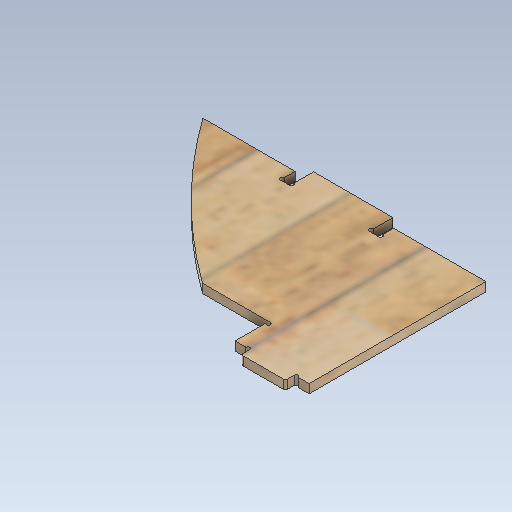
# Autodesk Inventor part: Support A1
Saved by Autodesk Inventor 2020 (Build 240168000, 168)
## iProperties
Created: 2020-03-07
Part Number: Support A1
Material: Wood (Maple)
Document SubType Name: Modeling
Designer: Daniel Wikman
Density: 0.67 g/cm^3
Appearance: Natural Maple - Glossy Dark Tint
Author: Daniel Wikman
Autodesk Inventor part; units mm, degrees
ref_plane "YZ Plane" through (0, 0, 0) normal (1, 0, 0) x (0, 1, 0)
ref_plane "XZ Plane" through (0, 0, 0) normal (0, 1, 0) x (-1, 0, 0)
ref_plane "XY Plane" through (0, 0, 0) normal (0, 0, 1) x (1, 0, 0)
sketch "Sketch1" plane through (0, 0, 0) normal (0, 1, 0) x (-1, 0, 0)
  arc A0 (-1.4864, -17.3614) -> (1.1787, -17.296) centre (-0.1546, -17.296) ccw
  arc A1 (31.1823, -17.2881) -> (33.847, -17.3614) centre (32.5157, -17.2881) ccw
  line L0 (33.847, -17.3614) -> (41.1803, -17.3614)
  line L1 (-1.4864, -17.3614) -> (-8.8197, -17.3614)
  line L2 (-8.8197, -17.3614) -> (-8.8197, -136.8614)
  line L3 (41.1803, -17.3614) -> (41.1803, -38.0281)
  arc A2 (41.1803, -38.0281) -> (40.0555, -40.0773) centre (40.0555, -38.7439) ccw
  line L4 (40.0555, -40.0773) -> (85.8888, -40.0773)
  line L5 (-8.8197, -136.8614) -> (53.5136, -136.8614)
  line L6 (53.5136, -136.8614) -> (53.5136, -129.5281)
  arc A3 (53.5136, -126.8614) -> (53.5136, -129.5281) centre (53.5136, -128.1947) ccw
  arc A4 (60.0136, -129.5281) -> (60.0136, -126.8614) centre (60.0136, -128.1947) ccw
  line L7 (60.0136, -129.5281) -> (60.0136, -142.8614)
  line L8 (60.0136, -126.8614) -> (53.5136, -126.8614)
  line L9 (120.137, -136.8614) -> (120.137, -129.5281)
  arc A5 (120.137, -129.5281) -> (120.137, -126.8614) centre (120.137, -128.1947) ccw
  arc A6 (113.637, -126.8614) -> (113.637, -129.5281) centre (113.637, -128.1947) ccw
  line L10 (113.637, -129.5281) -> (113.637, -142.8614)
  line L11 (113.637, -126.8614) -> (120.137, -126.8614)
  arc A7 (182.4703, -136.8614) -> (85.8888, -40.0773) centre (-162.7379, -384.7652) ccw
  line L12 (120.137, -136.8614) -> (182.4703, -136.8614)
  arc A8 (2.512, -11.3614) -> (1.1787, -12.6947) centre (2.512, -12.6947) ccw
  line L13 (1.1787, -12.6947) -> (1.1787, -17.296)
  arc A9 (31.1823, -12.6947) -> (29.849, -11.3614) centre (29.849, -12.6947) ccw
  line L14 (2.512, -11.3614) -> (29.849, -11.3614)
  line L15 (31.1823, -17.2881) -> (31.1823, -12.6947)
  line L16 (60.0136, -142.8614) -> (113.637, -142.8614)
  point P0 (0, 0)
  point P1 (28.8512, 3.0303)
  point P2 (-1.1488, 3.0309)
  dimension "d1" = 2.6667
  dimension "d2" = 30
  dimension "d4" = 2.6667
  dimension "d6" = 7.3333
  dimension "d7" = 7.3333
  dimension "d8" = 20.6667
  dimension "d9" = 2.6667
  dimension "d10" = 45.8333
  dimension "d11" = 119.5
  dimension "d12" = 62.3333
  dimension "d19" = 7.3333
  dimension "d53" = 2.6667
  dimension "d56" = 2.6667
  dimension "d58" = 6.5
  dimension "d59" = 13.3333
  dimension "d61" = 425
  dimension "d64" = 13.3333
  dimension "d67" = 7.3333
  dimension "d73" = 50
  dimension "d74" = 2.6667
  dimension "d75" = 6
  dimension "d76" = 191.29
  dimension "d77" = 6.5
  dimension "d78" = 6.5
  dimension "d79" = 6.5
  dimension "d80" = 1.3333
  dimension "d81" = 1.3333
  dimension "d82" = 90
  dimension "d83" = 2.6667
  dimension "d84" = 2.6667
  dimension "d85" = 2.6667
  dimension "d86" = 2.6667
  dimension "d87" = 53.6233
  constraints: 34 end point, 20 point on circle, 10 centre point, 8 horizontal, 8 tangent, 6 vertical, 3 collinear
  measures "d1" diameter of A0
  measures "d2" distance of point (28.851, 3.03) point (-1.149, 3.031)
  measures "d4" diameter of A1
  measures "d6" distance of L0.start L0.end
  measures "d7" distance of L1.start L1.end
  measures "d8" distance of L0.end L3.end
  measures "d9" diameter of A2
  measures "d10" distance of L4.start L4.end
  measures "d11" distance of L1.end L2.end
  measures "d12" distance of L2.end L5.end
  measures "d19" distance of L5.end L6.end
  measures "d53" diameter of A3
  measures "d56" diameter of A4
  measures "d58" distance between parallel lines of L6 L7
  measures "d59" distance of L7.start L7.end
  measures "d61" radius of A7
  measures "d64" distance of L10.start L10.end
  measures "d67" distance of L9.start L9.end
  measures "d73" distance between parallel lines of L2 L3
  measures "d74" diameter of A9
  measures "d75" distance between parallel lines of L0 L14
  measures "d76" distance from line of L12.end L2
  measures "d77" distance between parallel lines of L10 L9
  measures "d78" distance of L8.start L8.end
  measures "d79" distance of L11.start L11.end
  measures "d80" radius of A6
  measures "d81" radius of A5
  measures "d82" angle of L12 L9
  measures "d83" distance from line of L9.end L11
  measures "d84" distance from line of L10.start L11
  measures "d85" distance from line of L7.start L8
  measures "d86" distance of L6.end L8.end
  measures "d87" distance of L7.end L10.end
extrude "Extrusion1" add sketch "Sketch1" along normal blind 6
body "Solid1"
